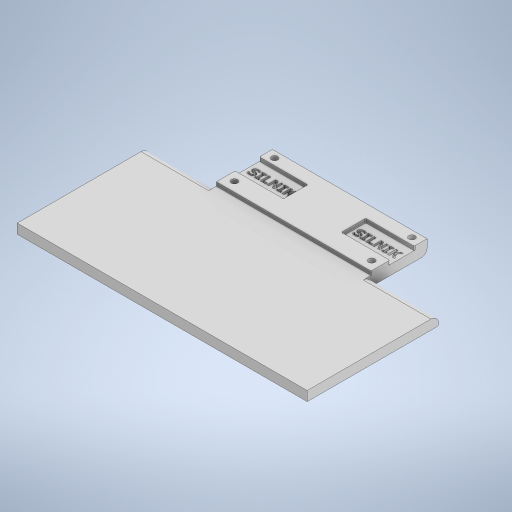
# Autodesk Inventor part: base
Saved by Autodesk Inventor 2023 (Build 270158000, 158)
## iProperties
Created: 2024-04-04
Part Number: base
Material: Ogólny
Document SubType Name: Modeling
Designer: Kamil
Density: 1 g/cm^3
Appearance: Domyślna
Author: Kamil
Autodesk Inventor part; units mm, degrees
ref_plane "YZ Plane" through (0, 0, 0) normal (1, 0, 0) x (0, 1, 0)
ref_plane "XZ Plane" through (0, 0, 0) normal (0, 1, 0) x (-1, 0, 0)
ref_plane "XY Plane" through (0, 0, 0) normal (0, 0, 1) x (1, 0, 0)
sketch "Szkic1" plane through (0, 0, 0) normal (0, 1, 0) x (-1, 0, 0)
  line L0 (75, -50) -> (-75, -50)
  line L1 (-75, -50) -> (-75, 50)
  line L2 (-75, 50) -> (75, 50)
  line L3 (75, 50) -> (75, -50)
  point P0 (0, 0)
  point P1 (0, -50)
  point P2 (-75, 0)
  dimension "d0" = 150
  dimension "d1" = 100
  constraints: 8 end point, 2 midpoint, 2 parallel, 1 horizontal, 1 horizontal alignment, 1 perpendicular, 1 vertical alignment
  measures "d0" distance of L1.end L2.end
  measures "d1" distance of L0.end L1.end
extrude "Wyciągnięcie proste1" add sketch "Szkic1" along normal blind 5
sketch "Szkic2" plane through (0, 5, 0) normal (0, 1, 0) x (1, 0, 0)
  line L0 (-75, -50) -> (75, -50) projected
  line L1 (75, -50) -> (75, 50) projected
  line L2 (75, 50) -> (-75, 50) projected
  line L3 (-75, 50) -> (-75, -50) projected
  line L4 (-75, 50) -> (-40, 50)
  line L5 (-40, 50) -> (-40, 18)
  line L6 (-40, 18) -> (-75, 18)
  line L7 (-75, 18) -> (-75, 50)
  line L8 (75, 50) -> (40, 50)
  line L9 (40, 50) -> (40, 18)
  line L10 (40, 18) -> (75, 18)
  line L11 (75, 18) -> (75, 50)
  point P0 (0, 0)
  point P1 (-57.5, 18)
  point P2 (57.5, 18)
  point P3 (75, 18)
  point P4 (-75, 18)
  dimension "d4" = 32
  dimension "d5" = 35
  dimension "d6" = 35
  constraints: 16 end point, 4 parallel, 2 horizontal, 2 midpoint, 2 perpendicular, 1 horizontal alignment, 1 point on line
  measures "d4" distance of L4.end L5.end
  measures "d5" distance of L2.end L4.end
  measures "d6" distance of L1.end L8.end
extrude "Wyciągnięcie proste2" cut sketch "Szkic2" against normal through all contours L3 L2 L5 L6 | L10 L9 L2 L1
sketch "Szkic3" plane through (0, 5, 0) normal (0, 1, 0) x (1, 0, 0)
  line L0 (40, 18) -> (40, 50) projected
  line L1 (40, 50) -> (-40, 50) projected
  line L2 (-40, 50) -> (-40, 18) projected
  line L3 (-40, 18) -> (-75, 18) projected
  line L4 (-75, 18) -> (-75, -50) projected
  line L5 (-75, -50) -> (75, -50) projected
  line L6 (75, -50) -> (75, 18) projected
  line L7 (75, 18) -> (40, 18) projected
  line L8 (40, 50) -> (-40, 50)
  line L9 (-40, 50) -> (-40, 47)
  line L10 (-40, 47) -> (40, 47)
  line L11 (40, 47) -> (40, 50)
  point P0 (0, 0)
  point P1 (40, 47)
  dimension "d9" = 3
  constraints: 8 end point, 2 parallel, 1 horizontal, 1 perpendicular, 1 point on line
  measures "d9" distance of L1.end L9.end
extrude "Wyciągnięcie proste3" cut sketch "Szkic3" against normal through all contours L10 L2 L1 L0
chamfer "Faza1" distance 2 angle 45 2 edges at (57.5, 5, -18) (-57.5, 5, -18)
fillet "Zaokrąglenie2" radius 4 4 edges at (57.5, 3, -18) (57.5, 5, -16) (-57.5, 3, -18) (-57.5, 5, -16)
sketch "Szkic4" plane through (0, 5, 0) normal (0, 1, 0) x (1, 0, 0)
  line L0 (-75, 14) -> (-40, 14) projected
  line L1 (-75, 14) -> (-75, -50) projected
  line L2 (-75, -50) -> (75, -50) projected
  line L3 (75, -50) -> (75, 14) projected
  line L4 (40, 14) -> (75, 14) projected
  line L5 (40, 14) -> (40, 47) projected
  line L6 (40, 47) -> (-40, 47) projected
  line L7 (-40, 47) -> (-40, 14) projected
  line L8 (40, 40.0002) -> (39.2, 40.0002) projected
  line L9 (39.2, 28.0002) -> (40, 28.0002) projected
  line L10 (-40, 44) -> (-40, 47) projected
  line L11 (40, 40.0002) -> (-40, 40.0002)
  line L12 (-40, 40.0002) -> (-40, 47)
  line L13 (-40, 47) -> (40, 47)
  line L14 (40, 47) -> (40, 40.0002)
  line L15 (-40, 18) -> (-40, 47) projected
  line L16 (40, 28.0002) -> (-40, 28.0002)
  line L17 (-40, 28.0002) -> (-40, 18.0002)
  line L18 (-40, 18.0002) -> (40, 18.0002)
  line L19 (40, 18.0002) -> (40, 28.0002)
  line L20 (15, 28.0002) -> (15, 18.0002)
  line L21 (-15, 18.0002) -> (-15, 28.0002)
  line L22 (40, 40.3002) -> (-40, 40.3002)
  line L23 (40, 47) -> (40, 18) projected
  line L24 (40, 27.7002) -> (-40, 27.7002)
  line L25 (-15, 18.0002) -> (-12, 18.0002)
  line L26 (-12, 40.3002) -> (-15, 40.3002)
  line L27 (-15, 40.3002) -> (-15, 18.0002)
  line L28 (15, 18.0002) -> (8, 18.0002)
  line L29 (8, 40.3002) -> (15, 40.3002)
  line L30 (15, 40.3002) -> (15, 18.0002)
  point P0 (0, 0)
  point P1 (15, 23.0002)
  point P2 (40, 44)
  point P3 (15, 27.7002)
  point P4 (-40, 40.3002)
  point P5 (-15, 27.7002)
  point P6 (-40, 27.7002)
  point P7 (-40, 18.0002)
  point P8 (40, 18.0002)
  dimension "d17" = 10
  dimension "d18" = 25
  dimension "d19" = 25
  dimension "d20" = 0.3
  dimension "d21" = 0.3
  constraints: 36 end point, 11 point on line, 6 parallel, 6 perpendicular, 4 horizontal, 2 vertical, 1 midpoint
  measures "d17" distance between parallel lines of L16 L18
  measures "d18" distance between parallel lines of L17 L21
  measures "d19" distance from line of L5 point (15, 23)
  measures "d20" distance between parallel lines of L16 L24
  measures "d21" distance between parallel lines of L22 L11
extrude "Wyciągnięcie proste4" add sketch "Szkic4" along normal blind 2 contours L7 L24 L21 L18 | L21 L24 L20 L18 | L21 L16 L20 L24 | L27 L11 L30 L16 | L24 L5 L18 L20 | L7 L6 L5 L22 | L27 L22 L30 L11
sketch "Szkic5" plane through (0, 5, 0) normal (0, 1, 0) x (1, 0, 0)
  line L0 (-15, 40.3002) -> (-40, 40.3002) projected
  line L1 (-40, 40.3002) -> (-40, 27.7002) projected
  line L2 (-40, 27.7002) -> (-15, 27.7002) projected
  line L3 (-15, 27.7002) -> (-15, 40.3002) projected
  line L4 (-38.5, 36.7502) -> (-15, 36.7502) construction
  line L5 (-15, 36.7502) -> (-15, 31.2502) construction
  line L6 (-15, 31.2502) -> (-38.5, 31.2502) construction
  line L7 (-38.5, 31.2502) -> (-38.5, 36.7502) construction
  line L8 (16, 36.7502) -> (39.5, 36.7502) construction
  line L9 (39.5, 36.7502) -> (39.5, 31.2502) construction
  line L10 (39.5, 31.2502) -> (16, 31.2502) construction
  line L11 (16, 31.2502) -> (16, 36.7502) construction
  line L12 (40, 27.7002) -> (40, 40.3002) projected
  spline S0 degree 2 poles (-36.6438, 31.67) (-37.1617, 31.67) (-37.9421, 31.8705) (-38.2776, 32.0164) knots 0 0 0 1 2 2 2
  line L13 (-38.2776, 32.0164) -> (-38.2776, 33.0885)
  line L14 (-38.2776, 33.0885) -> (-38.1754, 33.0885)
  spline S1 degree 2 poles (-38.1754, 33.0885) (-37.8363, 32.8005) (-37.0231, 32.4905) (-36.6402, 32.4905) knots 0 0 0 1 2 2 2
  spline S2 degree 2 poles (-36.6402, 32.4905) (-36.5417, 32.4905) (-36.2245, 32.5342) (-36.1297, 32.578) knots 0 0 0 1 2 2 2
  spline S3 degree 2 poles (-36.1297, 32.578) (-36.013, 32.6291) (-35.8489, 32.815) (-35.8489, 32.9646) knots 0 0 0 1 2 2 2
  spline S4 degree 2 poles (-35.8489, 32.9646) (-35.8489, 33.1359) (-36.1151, 33.3475) (-36.2974, 33.3949) knots 0 0 0 1 2 2 2
  spline S5 degree 2 poles (-36.2974, 33.3949) (-36.5271, 33.4569) (-37.0486, 33.5626) (-37.2784, 33.6428) knots 0 0 0 1 2 2 2
  spline S6 degree 2 poles (-37.2784, 33.6428) (-37.7998, 33.8252) (-38.252, 34.4487) (-38.252, 34.9155) knots 0 0 0 1 2 2 2
  spline S7 degree 2 poles (-38.252, 34.9155) (-38.252, 35.5464) (-37.1835, 36.3304) (-36.3813, 36.3304) knots 0 0 0 1 2 2 2
  spline S8 degree 2 poles (-36.3813, 36.3304) (-35.9801, 36.3304) (-35.1852, 36.1663) (-34.8716, 36.0278) knots 0 0 0 1 2 2 2
  line L15 (-34.8716, 36.0278) -> (-34.8716, 34.9994)
  line L16 (-34.8716, 34.9994) -> (-34.97, 34.9994)
  spline S9 degree 2 poles (-34.97, 34.9994) (-35.2216, 35.2146) (-35.9437, 35.5099) (-36.3229, 35.5099) knots 0 0 0 1 2 2 2
  spline S10 degree 2 poles (-36.3229, 35.5099) (-36.4724, 35.5099) (-36.7058, 35.4662) (-36.8371, 35.4078) knots 0 0 0 1 2 2 2
  spline S11 degree 2 poles (-36.8371, 35.4078) (-36.9429, 35.3604) (-37.096, 35.1708) (-37.096, 35.0541) knots 0 0 0 1 2 2 2
  spline S12 degree 2 poles (-37.096, 35.0541) (-37.096, 34.8791) (-36.8517, 34.6785) (-36.5016, 34.5983) knots 0 0 0 1 2 2 2
  spline S13 degree 2 poles (-36.5016, 34.5983) (-36.2755, 34.5472) (-35.8562, 34.4487) (-35.6155, 34.3649) knots 0 0 0 1 2 2 2
  spline S14 degree 2 poles (-35.6155, 34.3649) (-35.1487, 34.1935) (-34.6929, 33.6246) (-34.6929, 33.1578) knots 0 0 0 1 2 2 2
  spline S15 degree 2 poles (-34.6929, 33.1578) (-34.6929, 32.4868) (-35.7468, 31.67) (-36.6438, 31.67) knots 0 0 0 1 2 2 2
  line L17 (-31.874, 31.7502) -> (-34.2954, 31.7502)
  line L18 (-34.2954, 31.7502) -> (-34.2954, 32.5342)
  line L19 (-34.2954, 32.5342) -> (-33.6499, 32.5342)
  line L20 (-33.6499, 32.5342) -> (-33.6499, 35.4662)
  line L21 (-33.6499, 35.4662) -> (-34.2954, 35.4662)
  line L22 (-34.2954, 35.4662) -> (-34.2954, 36.2502)
  line L23 (-34.2954, 36.2502) -> (-31.874, 36.2502)
  line L24 (-31.874, 36.2502) -> (-31.874, 35.4662)
  line L25 (-31.874, 35.4662) -> (-32.5194, 35.4662)
  line L26 (-32.5194, 35.4662) -> (-32.5194, 32.5342)
  line L27 (-32.5194, 32.5342) -> (-31.874, 32.5342)
  line L28 (-31.874, 32.5342) -> (-31.874, 31.7502)
  line L29 (-28.1216, 31.7502) -> (-31.1228, 31.7502)
  line L30 (-31.1228, 31.7502) -> (-31.1228, 36.2502)
  line L31 (-31.1228, 36.2502) -> (-29.9923, 36.2502)
  line L32 (-29.9923, 36.2502) -> (-29.9923, 32.6072)
  line L33 (-29.9923, 32.6072) -> (-28.1216, 32.6072)
  line L34 (-28.1216, 32.6072) -> (-28.1216, 31.7502)
  line L35 (-23.7273, 31.7502) -> (-24.814, 31.7502)
  line L36 (-24.814, 31.7502) -> (-26.5498, 34.8864)
  line L37 (-26.5498, 34.8864) -> (-26.5498, 31.7502)
  line L38 (-26.5498, 31.7502) -> (-27.5818, 31.7502)
  line L39 (-27.5818, 31.7502) -> (-27.5818, 36.2502)
  line L40 (-27.5818, 36.2502) -> (-26.1961, 36.2502)
  line L41 (-26.1961, 36.2502) -> (-24.7593, 33.672)
  line L42 (-24.7593, 33.672) -> (-24.7593, 36.2502)
  line L43 (-24.7593, 36.2502) -> (-23.7273, 36.2502)
  line L44 (-23.7273, 36.2502) -> (-23.7273, 31.7502)
  line L45 (-20.5729, 31.7502) -> (-22.9943, 31.7502)
  line L46 (-22.9943, 31.7502) -> (-22.9943, 32.5342)
  line L47 (-22.9943, 32.5342) -> (-22.3489, 32.5342)
  line L48 (-22.3489, 32.5342) -> (-22.3489, 35.4662)
  line L49 (-22.3489, 35.4662) -> (-22.9943, 35.4662)
  line L50 (-22.9943, 35.4662) -> (-22.9943, 36.2502)
  line L51 (-22.9943, 36.2502) -> (-20.5729, 36.2502)
  line L52 (-20.5729, 36.2502) -> (-20.5729, 35.4662)
  line L53 (-20.5729, 35.4662) -> (-21.2184, 35.4662)
  line L54 (-21.2184, 35.4662) -> (-21.2184, 32.5342)
  line L55 (-21.2184, 32.5342) -> (-20.5729, 32.5342)
  line L56 (-20.5729, 32.5342) -> (-20.5729, 31.7502)
  line L57 (-15.8797, 31.7502) -> (-17.2472, 31.7502)
  line L58 (-17.2472, 31.7502) -> (-18.4688, 33.5772)
  line L59 (-18.4688, 33.5772) -> (-18.6912, 33.2709)
  line L60 (-18.6912, 33.2709) -> (-18.6912, 31.7502)
  line L61 (-18.6912, 31.7502) -> (-19.8217, 31.7502)
  line L62 (-19.8217, 31.7502) -> (-19.8217, 36.2502)
  line L63 (-19.8217, 36.2502) -> (-18.6912, 36.2502)
  line L64 (-18.6912, 36.2502) -> (-18.6912, 34.2409)
  line L65 (-18.6912, 34.2409) -> (-17.2472, 36.2502)
  line L66 (-17.2472, 36.2502) -> (-15.9453, 36.2502)
  line L67 (-15.9453, 36.2502) -> (-17.5498, 34.1607)
  line L68 (-17.5498, 34.1607) -> (-15.8797, 31.7502)
  spline S16 degree 2 poles (17.8562, 31.67) (17.3383, 31.67) (16.5579, 31.8705) (16.2224, 32.0164) knots 0 0 0 1 2 2 2
  line L69 (16.2224, 32.0164) -> (16.2224, 33.0885)
  line L70 (16.2224, 33.0885) -> (16.3246, 33.0885)
  spline S17 degree 2 poles (16.3246, 33.0885) (16.6637, 32.8005) (17.4769, 32.4905) (17.8598, 32.4905) knots 0 0 0 1 2 2 2
  spline S18 degree 2 poles (17.8598, 32.4905) (17.9583, 32.4905) (18.2755, 32.5342) (18.3703, 32.578) knots 0 0 0 1 2 2 2
  spline S19 degree 2 poles (18.3703, 32.578) (18.487, 32.6291) (18.6511, 32.815) (18.6511, 32.9646) knots 0 0 0 1 2 2 2
  spline S20 degree 2 poles (18.6511, 32.9646) (18.6511, 33.1359) (18.3849, 33.3475) (18.2026, 33.3949) knots 0 0 0 1 2 2 2
  spline S21 degree 2 poles (18.2026, 33.3949) (17.9729, 33.4569) (17.4514, 33.5626) (17.2216, 33.6428) knots 0 0 0 1 2 2 2
  spline S22 degree 2 poles (17.2216, 33.6428) (16.7002, 33.8252) (16.248, 34.4487) (16.248, 34.9155) knots 0 0 0 1 2 2 2
  spline S23 degree 2 poles (16.248, 34.9155) (16.248, 35.5464) (17.3165, 36.3304) (18.1187, 36.3304) knots 0 0 0 1 2 2 2
  spline S24 degree 2 poles (18.1187, 36.3304) (18.5199, 36.3304) (19.3148, 36.1663) (19.6284, 36.0278) knots 0 0 0 1 2 2 2
  line L71 (19.6284, 36.0278) -> (19.6284, 34.9994)
  line L72 (19.6284, 34.9994) -> (19.53, 34.9994)
  spline S25 degree 2 poles (19.53, 34.9994) (19.2784, 35.2146) (18.5563, 35.5099) (18.1771, 35.5099) knots 0 0 0 1 2 2 2
  spline S26 degree 2 poles (18.1771, 35.5099) (18.0276, 35.5099) (17.7942, 35.4662) (17.6629, 35.4078) knots 0 0 0 1 2 2 2
  spline S27 degree 2 poles (17.6629, 35.4078) (17.5571, 35.3604) (17.404, 35.1708) (17.404, 35.0541) knots 0 0 0 1 2 2 2
  spline S28 degree 2 poles (17.404, 35.0541) (17.404, 34.8791) (17.6483, 34.6785) (17.9984, 34.5983) knots 0 0 0 1 2 2 2
  spline S29 degree 2 poles (17.9984, 34.5983) (18.2245, 34.5472) (18.6438, 34.4487) (18.8845, 34.3649) knots 0 0 0 1 2 2 2
  spline S30 degree 2 poles (18.8845, 34.3649) (19.3513, 34.1935) (19.8071, 33.6246) (19.8071, 33.1578) knots 0 0 0 1 2 2 2
  spline S31 degree 2 poles (19.8071, 33.1578) (19.8071, 32.4868) (18.7532, 31.67) (17.8562, 31.67) knots 0 0 0 1 2 2 2
  line L73 (22.626, 31.7502) -> (20.2046, 31.7502)
  line L74 (20.2046, 31.7502) -> (20.2046, 32.5342)
  line L75 (20.2046, 32.5342) -> (20.8501, 32.5342)
  line L76 (20.8501, 32.5342) -> (20.8501, 35.4662)
  line L77 (20.8501, 35.4662) -> (20.2046, 35.4662)
  line L78 (20.2046, 35.4662) -> (20.2046, 36.2502)
  line L79 (20.2046, 36.2502) -> (22.626, 36.2502)
  line L80 (22.626, 36.2502) -> (22.626, 35.4662)
  line L81 (22.626, 35.4662) -> (21.9806, 35.4662)
  line L82 (21.9806, 35.4662) -> (21.9806, 32.5342)
  line L83 (21.9806, 32.5342) -> (22.626, 32.5342)
  line L84 (22.626, 32.5342) -> (22.626, 31.7502)
  line L85 (26.3784, 31.7502) -> (23.3772, 31.7502)
  line L86 (23.3772, 31.7502) -> (23.3772, 36.2502)
  line L87 (23.3772, 36.2502) -> (24.5077, 36.2502)
  line L88 (24.5077, 36.2502) -> (24.5077, 32.6072)
  line L89 (24.5077, 32.6072) -> (26.3784, 32.6072)
  line L90 (26.3784, 32.6072) -> (26.3784, 31.7502)
  line L91 (30.7727, 31.7502) -> (29.686, 31.7502)
  line L92 (29.686, 31.7502) -> (27.9502, 34.8864)
  line L93 (27.9502, 34.8864) -> (27.9502, 31.7502)
  line L94 (27.9502, 31.7502) -> (26.9182, 31.7502)
  line L95 (26.9182, 31.7502) -> (26.9182, 36.2502)
  line L96 (26.9182, 36.2502) -> (28.3039, 36.2502)
  line L97 (28.3039, 36.2502) -> (29.7407, 33.672)
  line L98 (29.7407, 33.672) -> (29.7407, 36.2502)
  line L99 (29.7407, 36.2502) -> (30.7727, 36.2502)
  line L100 (30.7727, 36.2502) -> (30.7727, 31.7502)
  line L101 (33.9271, 31.7502) -> (31.5057, 31.7502)
  line L102 (31.5057, 31.7502) -> (31.5057, 32.5342)
  line L103 (31.5057, 32.5342) -> (32.1511, 32.5342)
  line L104 (32.1511, 32.5342) -> (32.1511, 35.4662)
  line L105 (32.1511, 35.4662) -> (31.5057, 35.4662)
  line L106 (31.5057, 35.4662) -> (31.5057, 36.2502)
  line L107 (31.5057, 36.2502) -> (33.9271, 36.2502)
  line L108 (33.9271, 36.2502) -> (33.9271, 35.4662)
  line L109 (33.9271, 35.4662) -> (33.2816, 35.4662)
  line L110 (33.2816, 35.4662) -> (33.2816, 32.5342)
  line L111 (33.2816, 32.5342) -> (33.9271, 32.5342)
  line L112 (33.9271, 32.5342) -> (33.9271, 31.7502)
  line L113 (38.6203, 31.7502) -> (37.2528, 31.7502)
  line L114 (37.2528, 31.7502) -> (36.0312, 33.5772)
  line L115 (36.0312, 33.5772) -> (35.8088, 33.2709)
  line L116 (35.8088, 33.2709) -> (35.8088, 31.7502)
  line L117 (35.8088, 31.7502) -> (34.6783, 31.7502)
  line L118 (34.6783, 31.7502) -> (34.6783, 36.2502)
  line L119 (34.6783, 36.2502) -> (35.8088, 36.2502)
  line L120 (35.8088, 36.2502) -> (35.8088, 34.2409)
  line L121 (35.8088, 34.2409) -> (37.2528, 36.2502)
  line L122 (37.2528, 36.2502) -> (38.5547, 36.2502)
  line L123 (38.5547, 36.2502) -> (36.9502, 34.1607)
  line L124 (36.9502, 34.1607) -> (38.6203, 31.7502)
  point P0 (0, 0)
  point P1 (-38.5, 34.0002)
  point P2 (-40, 34.0002)
  point P3 (16, 34.0002)
  point P4 (39.5, 34.0002)
  dimension "d25" = 1.5
  dimension "d26" = 5.5
  dimension "d27" = 23.5
  dimension "d28" = 5.5
  dimension "d29" = 23.5
  dimension "d30" = 0.5
  constraints: 4 midpoint, 2 horizontal alignment, 4 other
  measures "d25" distance between parallel lines of L1 L7
  measures "d26" distance of L6.end L4.start
  measures "d27" distance of L5.end L6.end
  measures "d28" distance of L11.start L11.end
  measures "d29" distance of L9.end L11.start
  measures "d30" distance between parallel lines of L12 L9
extrude "Wyciągnięcie proste5" cut sketch "Szkic5" against normal blind 1.5 contours S0 L13 L14 S1 S2 S3 S4 S5 S6 S7 S8 L15 L16 S9 S10 S11 S12 S13 S14 S15 | L17 L18 L19 L20 L21 L22 L23 L24 L25 L26 L27 L28 | L29 L30 L31 L32 L33 L34 | L35 L36 L37 L38 L39 L40 L41 L42 L43 L44 | L45 L46 L47 L48 L49 L50 L51 L52 L53 L54 L55 L56 | L57 L58 L59 L60 L61 L62 L63 L64 L65 L66 L67 L68 | S16 L69 L70 S17 S18 S19 S20 S21 S22 S23 S24 L71 L72 S25 S26 S27 S28 S29 S30 S31 | L73 L74 L75 L76 L77 L78 L79 L80 L81 L82 L83 L84 | L85 L86 L87 L88 L89 L90 | L91 L92 L93 L94 L95 L96 L97 L98 L99 L100 | L101 L102 L103 L104 L105 L106 L107 L108 L109 L110 L111 L112 | L113 L114 L115 L116 L117 L118 L119 L120 L121 L122 L123 L124
sketch "Szkic6" plane through (0, 0, 0) normal (0, -1, 0) x (1, 0, 0)
  circle A0 centre (35.5, -43.65) radius 1.95 projected
  circle A1 centre (35.5, -22.85) radius 1.95 projected
  circle A2 centre (-35.5, -22.85) radius 1.95 projected
  circle A3 centre (-35.5, -43.65) radius 1.95 projected
  point P0 (0, 0)
hole "Otwór1" at (35.5, 0, -22.85) at (35.5, 0, -43.65) at (-35.5, 0, -43.65) at (-35.5, 0, -22.85) direction (0, 1, 0) diameter 3.2 depth 8 countersink diameter 6 countersink angle 90
fillet "Zaokrąglenie3" radius 3 1 edges at (0, 0, -47)
fillet "Zaokrąglenie4" radius 1 2 edges at (-57.5, 0, -18) (57.5, 0, -18)
fillet "Zaokrąglenie5" radius 0.5 8 edges at (-15, 6, -40.3002) (-15, 6, -27.7002) (15, 6, -40.3002) (15, 6, -27.7002) (-40, 6, -40.3002) (-40, 6, -27.7002) (40, 6, -40.3002) (40, 6, -27.7002)
